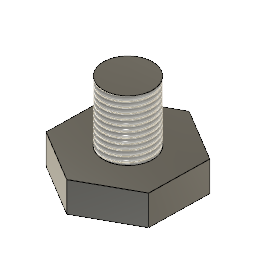
Nail v1 (Autodesk Fusion 360 design; units mm, degrees)
Autodesk Fusion 360 part; units mm, degrees
sketch "Sketch1" plane through (0, 0, 0) normal (0, 0, 1) x (1, 0, 0)
  line L0 (-34.3393, 20.6317) -> (-35.0372, -19.4228)
  line L1 (-35.0372, -19.4228) -> (-0.698, -40.0546)
  line L2 (-0.698, -40.0546) -> (34.3393, -20.6317)
  line L3 (34.3393, -20.6317) -> (35.0372, 19.4228)
  line L4 (35.0372, 19.4228) -> (0.698, 40.0546)
  line L5 (0.698, 40.0546) -> (-34.3393, 20.6317)
extrude "Extrude1" add sketch "Sketch1" along normal blind 20 makes body 1
sketch "Sketch2" plane through (0, 0, 20) normal (0, 0, 1) x (-1, 0, 0)
  line L0 (-0.698, -40.0546) -> (34.3393, -20.6317)
  line L1 (34.3393, -20.6317) -> (35.0372, 19.4228)
  line L2 (35.0372, 19.4228) -> (0.698, 40.0546)
  line L3 (0.698, 40.0546) -> (-34.3393, 20.6317)
  line L4 (-34.3393, 20.6317) -> (-35.0372, -19.4228)
  line L5 (-35.0372, -19.4228) -> (-0.698, -40.0546)
  circle A0 centre (0, 0) radius 16.161
  constraint coincident A0.centre origin
extrude "Extrude2" cut sketch "Sketch2" against normal blind 60 contours A0 bodies 1
sketch "Sketch3" plane through (0, 0, 0) normal (0, 0, 1) x (1, 0, 0)
  circle A0 centre (-100, 0) radius 16.6427
extrude "Extrude3" add sketch "Sketch3" along normal blind 50 separate body makes body 2
thread "Thread1" "ISO Metric profile 33.0 M33x3.5 6g" major diameter 32.7555 minor diameter 28.7529 pitch 3.5 angle 60 resizes the face on face at (-83.44, -1.6571, 16.6667) on bodies 2
move_body "Move1" bodies 2 to x (1, 0, 0) y (0, 1, 0) z (0, 0, 1) at (100, 0, 10)
combine "Combine1" operation add target body 1 tool bodies 2
thread "Thread2" "ISO Metric profile 33.0 M33x3.5 6g" major diameter 32.7555 minor diameter 28.7529 pitch 3.5 angle 60 resizes the face on face at (16.3574, 0.8164, 33.3333) on bodies 1
